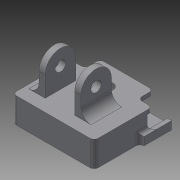
# Autodesk Inventor part: PulleyHolder
Saved by Autodesk Inventor 2013 (Build 170138000, 138)
## iProperties
Created: 2013-11-09
Part Number: PulleyHolder
Material: Generic
Document SubType Name: Modeling
Designer: JustinIndra
Density: 1 g/cm^3
Author: JustinIndra
Autodesk Inventor part; units mm, degrees
ref_plane "YZ Plane" through (0, 0, 0) normal (1, 0, 0) x (0, 1, 0)
ref_plane "XZ Plane" through (0, 0, 0) normal (0, 1, 0) x (-1, 0, 0)
ref_plane "XY Plane" through (0, 0, 0) normal (0, 0, 1) x (1, 0, 0)
sketch "Sketch1" plane through (0, 0, 0) normal (0, 1, 0) x (-1, 0, 0)
  line L0 (20, 0) -> (-20, 0)
  line L1 (-20, 0) -> (-20, 10)
  line L2 (-20, 10) -> (20, 10)
  line L3 (20, 10) -> (20, 0)
  circle A0 centre (0, 0) radius 3.175
  arc A1 (-20, 0) -> (20, 0) centre (0, 16.3026) ccw
  line L4 (20, 0) -> (-20, 0)
  line L5 (13.2784, -9.5) -> (-17.2645, -9.5) construction
  line L6 (20, 10) -> (-20, 10)
  line L7 (-20, 10) -> (-20, -10)
  line L8 (-20, -10) -> (20, -10)
  line L9 (20, -10) -> (20, 10)
  dimension "d0" = 40
  dimension "d2" = 6.35
  dimension "d4" = 9.5
  dimension "d5" = 10
  dimension "d6" = 20
  constraints: 20 end point, 5 parallel, 3 coincident, 3 perpendicular, 2 centre point, 2 horizontal, 2 point on circle, 1 collinear, 1 midpoint, 1 tangent
  measures "d0" distance of L1.end L2.end
  measures "d2" diameter of A0
  measures "d4" distance between parallel lines of L5 L0
  measures "d5" distance of L0.end L1.end
  measures "d6" distance of L8.end L2.end
extrude "Extrusion1" add sketch "Sketch1" along normal mid plane 8.5 contours L9 L8 L7 A1
sketch "Sketch2" plane through (0, -4.25, 0) normal (0, -1, 0) x (1, 0, 0)
  line L0 (20, -10) -> (20, 0) projected
  line L1 (-20, -10) -> (20, -10)
  line L2 (20, -10) -> (20, 10)
  line L3 (20, 10) -> (-20, 10)
  line L4 (-20, 10) -> (-20, -10)
  point P0 (0, 0)
  dimension "d9" = 20
  constraints: 8 end point, 2 parallel, 1 collinear, 1 horizontal, 1 perpendicular
  measures "d9" distance of L3.end L1.start
extrude "Extrusion2" add sketch "Sketch2" along normal blind 2
sketch "Sketch4" plane through (0, -4.25, 0) normal (0, 1, 0) x (1, 0, 0)
  circle A0 centre (0, 0) radius 3.175
  dimension "d12" = 6.35
  constraints: 1 centre point, 1 coincident
  measures "d12" diameter of A0
extrude "Extrusion3" cut sketch "Sketch4" against normal through all
mirror "Mirror1" about plane through (0, 0, 0) normal (0, 1, 0) of "Extrusion2", "Extrusion3"
sketch "Sketch5" plane through (0, -6.25, 0) normal (0, -1, 0) x (1, 0, 0)
  line L0 (-20, -10) -> (20, -10) projected
  line L1 (-20, 10) -> (-13, 10)
  line L2 (-13, 10) -> (-13, 2.5)
  line L3 (-13, 2.5) -> (-20, 2.5)
  line L4 (-20, 2.5) -> (-20, 10)
  dimension "d15" = 7
  dimension "d17" = 12.5
  constraints: 8 end point, 2 parallel, 1 horizontal, 1 perpendicular
  measures "d15" distance of L2.end L3.end
  measures "d17" distance between parallel lines of L3 L0
extrude "Extrusion4" cut sketch "Sketch5" against normal up to next
mirror "Mirror2" about plane through (0, 0, 0) normal (1, 0, 0) of "Extrusion4"
sketch "Sketch6" plane through (20, -6.25, -10) normal (0, 0, -1) x (-1, 0, 0)
  line L0 (40, 0) -> (40, 12.5) projected
  line L1 (0, 0) -> (40, 0)
  line L2 (40, 0) -> (40, 12.5)
  line L3 (40, 12.5) -> (0, 12.5)
  line L4 (0, 12.5) -> (0, 0)
  point P0 (20, 6.25)
  dimension "d20" = 12.5
  constraints: 8 end point, 2 parallel, 1 horizontal, 1 perpendicular, 1 point on line
  measures "d20" distance of L3.end L1.start
extrude "Extrusion5" add sketch "Sketch6" along normal blind 16
sketch "Sketch7" plane through (0, -6.25, 0) normal (0, -1, 0) x (1, 0, 0)
  circle A0 centre (0, 0) radius 3.175 projected
  line L0 (-13, -5) -> (-10, -5)
  line L1 (-10, -5) -> (-10, -20)
  line L2 (-10, -20) -> (-13, -20)
  line L3 (-13, -20) -> (-13, -5)
  line L4 (4.5, -5) -> (7.5, -5)
  line L5 (7.5, -5) -> (7.5, -20)
  line L6 (7.5, -20) -> (4.5, -20)
  line L7 (4.5, -20) -> (4.5, -5)
  dimension "d23" = 15
  dimension "d25" = 3
  dimension "d27" = 5
  dimension "d28" = 14.5
  dimension "d38" = 4.5
  constraints: 16 end point, 4 parallel, 2 equal length, 2 horizontal, 2 perpendicular, 1 collinear
  measures "d23" distance of L2.end L0.start
  measures "d25" distance of L1.end L2.end
  measures "d27" distance from line of A0.centre L0
  measures "d28" distance between parallel lines of L1 L7
  measures "d38" distance from line of L7 A0.centre
extrude "Extrusion6" add sketch "Sketch7" along normal blind 17.5 contours L0 L1 L2 L3 | L4 L5 L6 L7
sketch "Sketch8" plane through (-13, -6.25, -20) normal (-1, 0, 0) x (0, 0, 1)
  line L0 (15, -17.5) -> (0, -17.5) projected
  circle A0 centre (7.5, -10) radius 2.55
  point P0 (20, 6.25)
  point P1 (7.5, -17.5)
  dimension "d31" = 5.1
  dimension "d34" = 7.5
  constraints: 1 centre point, 1 midpoint, 1 vertical alignment
  measures "d31" diameter of A0
  measures "d34" distance from line of L0 A0.centre
extrude "Extrusion7" cut sketch "Sketch8" against normal through all
fillet "Fillet1" radius 7.5 4 edges at (6, -23.75, -5) (-11.5, -23.75, -5) (-11.5, -23.75, -20) (6, -23.75, -20)
fillet "Fillet2" radius 5 2 edges at (7.5, -6.25, -12.5) (-13, -6.25, -12.5)
fillet "Fillet3" radius 2 8 edges at (13, -5.25, 2.5) (-13, -5.25, 2.5) (-13, -5.25, 10) (13, -5.25, 10) (-20, -5.25, 2.5) (20, -5.25, 2.5) (20, 0, -26) (-20, 0, -26)
sketch "Sketch9" plane through (0, 4.25, 16.3026) normal (0, -1, 0) x (1, 0, 0)
  line L0 (-20, -6.3026) -> (-22, -6.3026)
  line L1 (-22, -6.3026) -> (-22, -19.8026)
  line L2 (-22, -19.8026) -> (-20, -19.8026)
  line L3 (-20, -19.8026) -> (-20, -6.3026)
  dimension "d41" = 2
  dimension "d42" = 13.5
  constraints: 8 end point, 2 parallel, 1 horizontal, 1 perpendicular
  measures "d41" distance of L0.start L0.end
  measures "d42" distance of L0.end L1.end
extrude "Extrusion8" add sketch "Sketch9" along normal mid plane 4
mirror "Mirror3" about plane through (0, 0, 0) normal (1, 0, 0) of "Extrusion8"
fillet "Fillet4" radius 2 4 edges at (-20, 4.25, -3.5) (-20, 2.25, -1.75) (20, 2.25, -1.75) (20, 4.25, -3.5)
equation "\"d6\" = 2 * d5"
body "Solid1"
